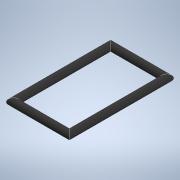
# Autodesk Inventor part: Rubber Seal
Saved by Autodesk Inventor 2022 (Build 260153000, 153)
## iProperties
Created: 2021-11-09
Part Number: Rubber Seal
Material: Rubber, Silicone
Document SubType Name: Modeling
Designer: Caleb
Density: 1.25 g/cm^3
Appearance: Rubber - Black
Author: Caleb
Autodesk Inventor part; units mm, degrees
ref_plane "YZ Plane" through (0, 0, 0) normal (1, 0, 0) x (0, 1, 0)
ref_plane "XZ Plane" through (0, 0, 0) normal (0, 1, 0) x (-1, 0, 0)
ref_plane "XY Plane" through (0, 0, 0) normal (0, 0, 1) x (1, 0, 0)
sketch "Sketch1" plane through (0, 0, 0) normal (0, 1, 0) x (-1, 0, 0)
  line L0 (-10.1905, -17.6905) -> (10.1905, -17.6905)
  line L1 (10.1905, -17.6905) -> (10.1905, 17.6905)
  line L2 (10.1905, 17.6905) -> (-10.1905, 17.6905)
  line L3 (-10.1905, 17.6905) -> (-10.1905, -17.6905)
  line L4 (-10.1905, -17.6905) -> (10.1905, 17.6905) construction
  line L5 (10.1905, -17.6905) -> (-10.1905, 17.6905) construction
  point P0 (0, 0)
  dimension "d0" = 35.381
  dimension "d1" = 20.381
  constraints: 12 end point, 2 midpoint, 2 parallel, 1 horizontal, 1 perpendicular
  measures "d0" distance of L0.end L1.end
  measures "d1" distance of L1.end L2.end
sketch "Sketch2" plane through (0, 0, 0) normal (0, 0, 1) x (1, 0, 0)
  circle A0 centre (10.1905, 0) radius 1.3081
  point P0 (0, 0)
  point P1 (10.1905, 0)
  dimension "d2" = 2.6162
  constraints: 1 centre point, 1 coincident
  measures "d2" diameter of A0
sweep "Sweep1" add profiles "Sketch2" path "Sketch1" path curves L3 L0 L1 L2
body "Solid1"
